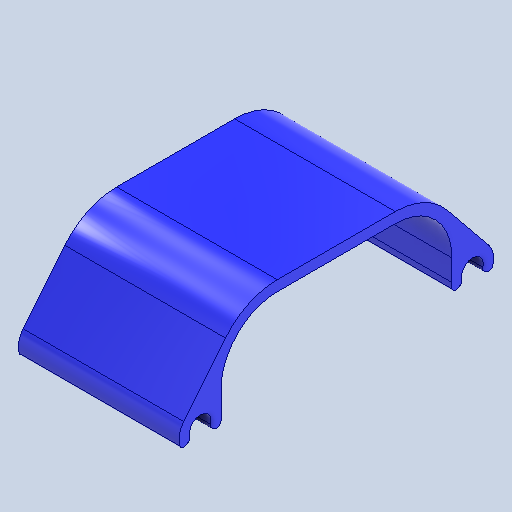
# Autodesk Inventor part: base_weel-v3-3DP-3
Saved by Autodesk Inventor 2025.2 (Build 292293000, 293)
## iProperties
Created: 2025-04-13
Part Number: base_weel-v3-3DP-3
Material: ABS プラスチック
Document SubType Name: Modeling
Designer: haruy
Density: 1.06 g/cm^3
Appearance: 青 - 壁塗料 - 光沢
Author: haruy
Autodesk Inventor part; units mm, degrees
ref_plane "YZ Plane" through (0, 0, 0) normal (1, 0, 0) x (0, 1, 0)
ref_plane "XZ Plane" through (0, 0, 0) normal (0, 1, 0) x (-1, 0, 0)
ref_plane "XY Plane" through (0, 0, 0) normal (0, 0, 1) x (1, 0, 0)
derived "base_weel-v3-Plate-1.ipt"
sketch "スケッチ1" plane through (0, 0, 0) normal (1, 0, 0) x (0, 1, 0)
  line L0 (0, 0) -> (20, 0)
  line L1 (20, 0) -> (20, -110)
  line L2 (20, -110) -> (0, -110)
  line L3 (0, -110) -> (0, 0)
  circle A0 centre (40, -55) radius 52.5
  line L4 (-12.5, 72.5213) -> (-12.5, -343.3137)
  circle A1 centre (40, -55) radius 9.5 construction
  circle A2 centre (40, -55) radius 20
  circle A3 centre (68.2843, -26.7157) radius 20
  circle A4 centre (68.2843, -83.2843) radius 20
  line L5 (68.2843, -26.7157) -> (40, -55)
  line L6 (40, -55) -> (68.2843, -83.2843)
  line L7 (40, -55) -> (40, -2.5)
  line L8 (0, 15) -> (20, 15)
  line L9 (20, 15) -> (20, -125)
  line L10 (20, -125) -> (0, -125)
  line L11 (0, -125) -> (0, 15)
  circle A5 centre (68.2843, -26.7157) radius 23.5
  circle A6 centre (57.4091, 10.2164) radius 5
  circle A7 centre (57.4091, -120.2164) radius 5
  line L12 (20, -20) -> (0, -20)
  line L13 (0, -55) -> (20, -55)
  circle A8 centre (40, -55) radius 9
  circle A9 centre (57.4091, 10.2164) radius 1.5
  circle A10 centre (57.4091, -120.2164) radius 1.5
  line L14 (20, -20) -> (53.8799, 13.7583)
  line L15 (62.4057, 10.0326) -> (59.9865, -55.7352)
  circle A11 centre (10, -55) radius 1.25
  circle A12 centre (10, -35) radius 1.25
  line L16 (62.4057, -120.0326) -> (59.9865, -54.2648)
  line L17 (20, -90) -> (53.8799, -123.7583)
  circle A13 centre (10, -75) radius 1.25
  line L18 (20, -90) -> (0, -90)
  circle A14 centre (68.2843, -26.7157) radius 22
  circle A15 centre (68.2843, -26.7157) radius 27
  circle A16 centre (68.2843, -83.2843) radius 22 construction
  circle A17 centre (57.4091, 10.2164) radius 5.2
  line L19 (57.4091, 10.2164) -> (57.4091, 15.4164)
  line L20 (57.4091, 10.2164) -> (54.8091, 14.7197)
  line L21 (57.4091, 10.2164) -> (57.4091, 5.0164)
  line L22 (57.4091, 10.2164) -> (54.8091, 5.713)
  line L23 (40, -55) -> (20, -55)
  circle A18 centre (57.4091, -120.2164) radius 5.2
  line L24 (57.4091, -120.2164) -> (54.8091, -124.7197)
  line L25 (57.4091, -120.2164) -> (54.8091, -115.713)
  circle A19 centre (57.4091, 10.2164) radius 10.2
  line L26 (64.9557, 17.0785) -> (88.2607, -8.5514) construction
  line L27 (54.8091, 14.7197) -> (52.3091, 19.0498)
  line L28 (54.8091, 5.713) -> (52.3091, 1.3829)
  line L29 (52.3091, 1.3829) -> (57.8472, -1.8146) construction
  line L30 (57.8472, -1.8146) -> (63.7063, -5.1973) construction
  circle A20 centre (57.4091, -120.2164) radius 10.2
  line L31 (64.9557, -127.0785) -> (88.2607, -101.4486) construction
  line L32 (54.8091, -124.7197) -> (52.3091, -129.0498)
  line L33 (54.8091, -115.713) -> (52.3091, -111.3829)
  line L34 (52.3091, -111.3829) -> (57.8472, -108.1854) construction
  line L35 (57.8472, -108.1854) -> (63.7063, -104.8027) construction
  circle A21 centre (68.2843, -83.2843) radius 27
  circle A22 centre (40, -55) radius 57.5 construction
  circle A23 centre (40, -55) radius 62.5 construction
  line L36 (94.026, -18.5694) -> (99.5873, -36.1427) construction
  line L37 (94.026, -91.4306) -> (99.5873, -73.8573) construction
  circle A24 centre (68.2843, -26.7157) radius 27
  circle A25 centre (68.2843, -26.7157) radius 32
  circle A26 centre (68.2843, -83.2843) radius 32
  line L38 (63.8425, 18.1316) -> (88.4677, -1.8837)
  line L39 (57.6718, 0.0198) -> (67.5887, 0.2753)
  line L40 (100.2843, -26.7157) -> (100.2843, -83.2843)
  line L41 (95.2843, -26.7157) -> (95.2843, -83.2843)
  line L42 (63.8425, -128.1316) -> (88.4677, -108.1163)
  line L43 (57.6718, -110.0198) -> (67.5887, -110.2753)
  point P0 (95.2843, -26.7157)
  point P1 (95.2843, -83.2843)
  point P2 (90.2843, -26.7157)
  point P3 (90.2843, -83.2843)
  point P4 (63.7063, -104.8027)
  point P5 (88.2607, -101.4486)
  point P6 (61.8363, -4.1176)
  point P7 (61.8857, -4.1036)
  point P8 (61.8842, -4.1453)
  point P9 (62.0789, 1.1481)
  point P10 (62.3532, 8.6053)
  point P11 (60.2417, -48.7967)
  point P12 (60.1074, -52.4478)
  point P13 (62.02, -0.4525)
  point P14 (60.2999, -47.2157)
  point P15 (61.8275, -5.6845)
  point P16 (67.5887, 0.2753)
  point P17 (95.2843, -26.7157)
  point P18 (67.5887, -110.2753)
  point P19 (57.6718, -110.0198)
  point P20 (63.8425, -128.1316)
  point P21 (88.4677, -108.1163)
  dimension "d3" = 44
  dimension "d1" = 44
  dimension "d2" = 5
  dimension "d4" = 10.4
  dimension "d5" = 30
  dimension "d6" = 30
  dimension "d7" = 5
  dimension "d11" = 5
  dimension "d12" = 5
  dimension "d13" = 5
  dimension "d14" = 5
  dimension "d15" = 5
  measures "d1" diameter of A14
  measures "d2" radial gap between concentric circles of A14 A15
  measures "d4" diameter of A17
  measures "d7" radial gap between concentric circles of A17 A19
  measures "d13" radial gap between concentric circles of A14 A24
  measures "d14" radial gap between concentric circles of A24 A25
extrude "押し出し1" add sketch "スケッチ1" against normal blind 77 contours A19 A25 L15 A17 L27 | L28 A17 L15 A25 A19 | A25 L15 A19 | L38 A25 A19 | A26 L16 A18 L33 A20 | A20 L16 A26 | A19 L15 L39 | A25 A19 L15 | A25 L41 A15 L39 L15 A19 | L32 A18 L16 A26 A20 | L43 L16 A20 | L16 A20 A26 | L40 A26 L41 A25 | A20 A26 L42 | L43 A21 L41 A26 A20 L16
fillet "フィレット1" radius 2 8 edges at (-38.5, 52.3091, 19.0498) (-38.5, 54.8091, 14.7197) (-38.5, 54.8091, 5.713) (-38.5, 52.3091, 1.3829) (-38.5, 52.3091, -111.3829) (-38.5, 54.8091, -115.713) (-38.5, 54.8091, -124.7197) (-38.5, 52.3091, -129.0498)
equation "\"d6\" = d5"
